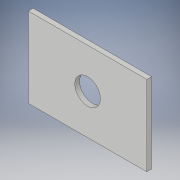
# Autodesk Inventor part: Back
Saved by Autodesk Inventor 2018 (Build 220112000, 112)
## iProperties
Created: 2018-04-18
Part Number: Back
Material: Generic
Document SubType Name: Modeling
Designer: trent
Density: 1 g/cm^3
Appearance: Default
Author: trent
Autodesk Inventor part; units mm, degrees
ref_plane "YZ Plane" through (0, 0, 0) normal (1, 0, 0) x (0, 1, 0)
ref_plane "XZ Plane" through (0, 0, 0) normal (0, 1, 0) x (-1, 0, 0)
ref_plane "XY Plane" through (0, 0, 0) normal (0, 0, 1) x (1, 0, 0)
sketch "Sketch1" plane through (0, 0, 0) normal (0, 0, 1) x (1, 0, 0)
  line L0 (-58.7375, -39.6875) -> (58.7375, -39.6875)
  line L1 (58.7375, -39.6875) -> (58.7375, 39.6875)
  line L2 (58.7375, 39.6875) -> (-58.7375, 39.6875)
  line L3 (-58.7375, 39.6875) -> (-58.7375, -39.6875)
  line L4 (-58.7375, -39.6875) -> (58.7375, 39.6875) construction
  line L5 (58.7375, -39.6875) -> (-58.7375, 39.6875) construction
  point P0 (0, 0)
  dimension "d0" = 117.475
  dimension "d1" = 79.375
  constraints: 12 end point, 2 midpoint, 2 parallel, 1 horizontal, 1 perpendicular
  measures "d0" distance of L2.end L1.end
  measures "d1" distance of L1.end L0.end
extrude "Extrusion1" add sketch "Sketch1" along normal blind 4.7625
sketch "Sketch2" plane through (0, 0, 4.7625) normal (0, 0, 1) x (1, 0, 0)
  circle A0 centre (0, 0) radius 12.7
  dimension "d4" = 25.4
  constraints: 1 centre point, 1 coincident
  measures "d4" diameter of A0
extrude "Extrusion2" cut sketch "Sketch2" against normal through all
body "Solid1"
